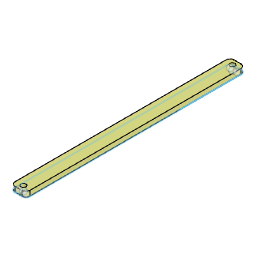
Very long Bar (Autodesk Fusion 360 design; units mm, degrees)
Autodesk Fusion 360 part; units mm, degrees
sketch "sketch 281" plane through (0, 0, 0) normal (0, 0, 1) x (1, 0, 0)
  circle A0 centre (7.5, 215) radius 2.5
  circle A1 centre (7.5, 5) radius 2.5
  arc A2 (15, 216) -> (11, 220) centre (11, 216) ccw
  line L0 (4, 220) -> (11, 220)
  arc A3 (4, 220) -> (0, 216) centre (4, 216) ccw
  line L1 (0, 4) -> (0, 216)
  arc A4 (0, 4) -> (4, 0) centre (4, 4) ccw
  line L2 (11, 0) -> (4, 0)
  arc A5 (11, 0) -> (15, 4) centre (11, 4) ccw
  line L3 (15, 216) -> (15, 4)
extrude "Extrude1" add sketch "sketch 281" along normal blind 5
